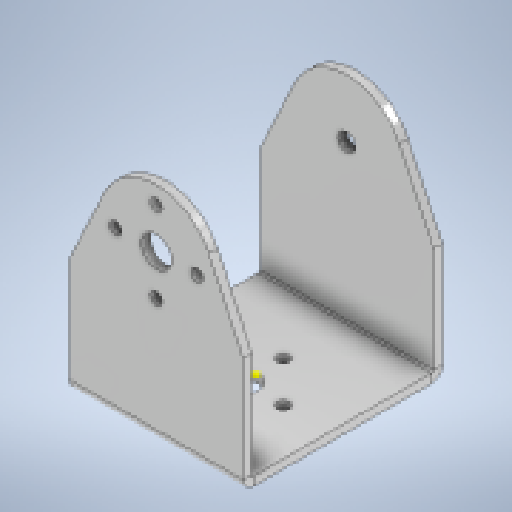
# Autodesk Inventor part: axis_7_top_frame
Saved by Autodesk Inventor 2025.2 (Build 292293000, 293)
## iProperties
Created: 2025-05-04
Part Number: axis_7_top_frame
Material: Aluminum 6061-AHC
Document SubType Name: Sheet Metal
Designer: User
Density: 2.7 g/cm^3
Sheet Metal Rule: Default_mm
Appearance: Aluminum - Dark
Author: User
Autodesk Inventor part; units mm, degrees
ref_plane "YZ Plane" through (0, 0, 0) normal (1, 0, 0) x (0, 1, 0)
ref_plane "XZ Plane" through (0, 0, 0) normal (0, 1, 0) x (-1, 0, 0)
ref_plane "XY Plane" through (0, 0, 0) normal (0, 0, 1) x (1, 0, 0)
sketch "Sketch1" plane through (0, 0, 0) normal (0, 1, 0) x (-1, 0, 0)
  line L0 (15, -15.715) -> (-15, -15.715)
  line L1 (-15, -15.715) -> (-15, 15.715)
  line L2 (-15, 15.715) -> (15, 15.715)
  line L3 (15, 15.715) -> (15, -15.715)
  point P0 (0, 0)
  dimension "d0" = 30
  dimension "d1" = 31.43
  dimension "d2" = 15
  dimension "d3" = 15.715
  measures "d0" distance of L0.start L0.end
  measures "d1" distance of L0.end L1.end
  measures "d2" distance from line of L3 point (0, 0)
  measures "d3" distance from line of point (0, 0) L0
extrude "Plate1" add sketch "Sketch1" along normal blind 1.5
sketch "Sketch2" plane through (15, 0, 17.215) normal (0, 0, -1) x (-1, 0, 0)
  line L0 (30, 0) -> (0, 0)
  line L1 (0, 0) -> (0, 40)
  line L2 (0, 40) -> (30, 40)
  line L3 (30, 40) -> (30, 0)
  constraints: 8 end point
edge flange "Flange1" height 40 angle 90 thickness 1.5 bend radius 0.31 thickness toward (0, 0, -1) relief straight relief width 1.5 relief depth 0.75 edges at (0, 1.5, 15.715) wall of the first edge with corners at (-15, 0, 17.215) (15, 0, 17.215) (15, 40, 17.215) (-15, 40, 17.215)
bend "Bend1"
corner "Corner1"
sketch "Sketch3" plane through (-15, 0, -17.215) normal (0, 0, 1) x (1, 0, 0)
  line L0 (30, 0) -> (0, 0)
  line L1 (0, 0) -> (0, 40)
  line L2 (0, 40) -> (30, 40)
  line L3 (30, 40) -> (30, 0)
  constraints: 8 end point
edge flange "Flange2" height 40 angle 90 thickness 1.5 bend radius 0.31 thickness toward (0, 0, 1) relief straight relief width 1.5 relief depth 0.75 edges at (0, 1.5, -15.715) wall of the first edge with corners at (15, 0, -17.215) (-15, 0, -17.215) (-15, 40, -17.215) (15, 40, -17.215)
bend "Bend2"
corner "Corner2"
sketch "Sketch6" plane through (-15, 40, 17.215) normal (0, 0, 1) x (1, 0, 0)
  circle A0 centre (15, -11.5) radius 10
  line L0 (5, -11.5) -> (5, 8.5)
  line L1 (5, 8.5) -> (25, 8.5)
  line L2 (25, 8.5) -> (25, -11.5)
  line L3 (0, 0) -> (30, 0) projected
  line L4 (0, -38.19) -> (0, 0) projected
  line L5 (5.9376, -7.2723) -> (0, -20)
  line L6 (24.0624, -7.2723) -> (30, -20)
  line L7 (30, -40) -> (0, -40) projected
  line L8 (30, 0) -> (30, -38.19) projected
  point P0 (15, -40)
  point P1 (5, -11.5)
  point P2 (25, -11.5)
  point P3 (25, 0)
  point P4 (5, -9.2822)
  point P5 (5, 0)
  point P6 (30, -20)
  point P7 (25, -9.2822)
  dimension "d39" = 28.5
  dimension "d40" = 20
  dimension "d41" = 20
  dimension "d42" = 20
  dimension "d43" = 20
  dimension "d45" = 15
  dimension "d48" = 20
  dimension "d49" = 20
  dimension "d50" = 0
  constraints: 6 end point, 4 point on circle, 2 tangent, 1 centre point, 1 horizontal, 1 point on line, 7 other
  measures "d39" distance of point (15, -40) A0.centre
  measures "d40" diameter of A0
  measures "d41" distance of A0.start L1.start
  measures "d42" distance of L1.start L1.end
  measures "d43" distance of L1.end A0.end
  measures "d45" distance from line of L4 A0.centre
  measures "d48" distance from line of L7 L5.end
  measures "d49" distance from line of L7 L6.end
  measures "d50" distance from line of L8 L6.end
extrude "Extrusion1" cut sketch "Sketch6" against normal blind 50 contours A0 L5 L0 L3 L2 L6 | L2 L3 L8 L6 | L5 L4 L3 L0
sketch "Sketch7" plane through (-15, 1.81, 17.215) normal (0, 0, 1) x (1, 0, 0)
  arc A0 (24.0624, 30.9177) -> (5.9376, 30.9177) centre (15, 26.69) ccw projected
  circle A1 centre (22, 26.69) radius 1.05
  circle A2 centre (15, 33.69) radius 1.05
  circle A3 centre (8, 26.69) radius 1.05
  circle A4 centre (15, 19.69) radius 1.05
  point P0 (15, -1.81)
  dimension "d51" = 7
  dimension "d52" = 2.1
  dimension "d55" = 360
  constraints: 4 centre point, 9 other
  measures "d51" distance of A0.centre A1.centre
  measures "d52" diameter of A1
extrude "Extrusion2" cut sketch "Sketch7" against normal blind 20
sketch "Sketch8" plane through (0, 1.5, 0) normal (0, 1, 0) x (1, 0, 0)
  line L0 (15, 15.715) -> (9.0624, 15.715) projected
  line L1 (9.0624, 15.715) -> (-9.0624, 15.715) projected
  line L2 (-9.0624, 15.715) -> (-15, 15.715) projected
  line L3 (-15, 15.715) -> (15, 15.715) projected
  circle A0 centre (0, -2.285) radius 2.6
  point P0 (0, 0)
  point P1 (7, -2.285)
  point P2 (0, 4.715)
  point P3 (-7, -2.285)
  point P4 (0, -9.285)
  dimension "d59" = 18
  dimension "d60" = 0
  dimension "d61" = 5.2
  dimension "d62" = 7
  dimension "d63" = 0
  dimension "d66" = 360
  constraints: 1 centre point, 5 other
  measures "d59" vertical distance of L2.end A0.centre
  measures "d60" horizontal distance of point (0, 0) A0.centre
  measures "d61" diameter of A0
  measures "d62" distance of A0.centre point (7, -2.285)
  measures "d63" vertical distance of A0.centre point (7, -2.285)
extrude "Extrusion3" cut sketch "Sketch8" against normal blind 10
sketch "Sketch9" plane through (0, 1.5, 0) normal (0, 1, 0) x (1, 0, 0)
  point P0 (0, 0)
hole "Hole3" at (0, 1.5, -4.715) at (7, 1.5, 2.285) at (-7, 1.5, 2.285) at (0, 1.5, 9.285) direction (0, -1, 0) diameter 2.1 depth 1.5
hole "Hole4" at (0, 28.5, 17.215) direction (0, 0, -1) diameter 5.2 depth 1.5 clearance for "Hex Head Bolt" size "M5" standard "Ansi Metric M Profile"
sketch "Sketch10" plane through (15, 1.81, -17.215) normal (0, 0, -1) x (-1, 0, 0)
  circle A0 centre (15, 26.69) radius 2.6 projected
  point P0 (15, -1.81)
hole "Hole5" at (0, 28.5, -17.215) direction (0, 0, 1) diameter 3 depth 1.5
equation "\"d75\" = Thickness"
equation "\"d82\" = Thickness"
equation "\"d89\" = Thickness"
equation "\"d4\" = Thickness"
equation "\"d5\" = BendReliefWidth"
equation "\"d6\" = BendReliefDepth"
equation "\"d7\" = MinimumRemnant"
equation "\"d8\" = TransitionRadius"
equation "\"d11\" = BendRadius"
equation "\"d12\" = CornerReliefSize"
equation "\"d13\" = GapSize"
equation "\"d14\" = JacobiRadiusSize"
equation "\"d15\" = BendReliefWidth"
equation "\"d16\" = BendReliefDepth"
equation "\"d17\" = MinimumRemnant"
equation "\"d18\" = TransitionRadius"
equation "\"d21\" = BendRadius"
equation "\"d22\" = CornerReliefSize"
equation "\"d23\" = GapSize"
equation "\"d24\" = JacobiRadiusSize"
equation "\"BendReliefWidth\" = Thickness"
equation "\"BendReliefDepth\" = 0.5 * Thickness"
equation "\"CornerReliefSize\" = 4 * Thickness"
equation "\"MinimumRemnant\" = 2 * Thickness"
equation "\"TransitionRadius\" = BendRadius"
equation "\"JacobiRadiusSize\" = BendRadius"
equation "\"GapSize\" = Thickness"
equation "\"Thickness\" = 1.5"
equation "\"BendRadius\" = 0.31"
body "Solid1"
